Autodesk Inventor part; units mm, degrees
(part 2 of 2)
sketch "スケッチ6" plane through (0, 0, 0) normal (0, 0, 1) x (1, 0, 0)
  arc A0 (-3.1442, 14.278) -> (-3.8445, 14.3466) centre (-3.5856, 13.3807) ccw projected
  arc A1 (-3.8445, 14.3466) -> (-4.7248, 14.0812) centre (0, 0) ccw projected
  arc A2 (-5.6301, 14.2199) -> (-4.7248, 14.0812) centre (-5.0429, 15.0293) ccw projected
  arc A3 (-5.6301, 14.2199) -> (-11.7841, 9.7488) centre (-7.979, 10.9821) ccw projected
  arc A4 (-11.932, 8.8449) -> (-11.7841, 9.7488) centre (-12.7354, 9.4404) ccw projected
  arc A5 (-11.932, 8.8449) -> (-12.4564, 8.0897) centre (0, 0) ccw projected
  arc A6 (-12.4564, 8.0897) -> (-12.6076, 7.4025) centre (-11.6178, 7.545) ccw projected
  arc A7 (-12.6076, 7.4025) -> (-11.6883, 4.5478) centre (-3.7583, 8.6769) ccw projected
  arc A8 (-12.1291, 3.191) -> (-11.6883, 4.5478) centre (-12.5752, 4.0859) ccw projected
  arc A9 (-12.1291, 3.191) -> (-14.5508, 1.4218) centre (-8.1406, -4.8107) ccw projected
  arc A10 (-14.5508, 1.4218) -> (-14.8325, 0.777) centre (-13.8338, 0.7247) ccw projected
  arc A11 (-14.8325, 0.777) -> (-14.8521, -0.1422) centre (0, 0) ccw projected
  arc A12 (-15.2637, -0.9604) -> (-14.8521, -0.1422) centre (-15.8521, -0.1518) ccw projected
  arc A13 (-15.2637, -0.9604) -> (-12.9131, -8.1948) centre (-12.9103, -4.1948) ccw projected
  arc A14 (-12.0992, -8.6148) -> (-12.9131, -8.1948) centre (-12.9138, -9.1948) ccw projected
  arc A15 (-12.0992, -8.6148) -> (-11.543, -9.3469) centre (0, 0) ccw projected
  arc A16 (-11.543, -9.3469) -> (-10.9361, -9.703) centre (-10.7658, -8.7176) ccw projected
  arc A17 (-10.9361, -9.703) -> (-7.9371, -9.7108) centre (-9.4136, -0.893) ccw projected
  arc A18 (-6.7829, -10.5494) -> (-7.9371, -9.7108) centre (-7.7719, -10.6971) ccw projected
  arc A19 (-6.7829, -10.5494) -> (-5.8487, -13.3993) centre (2.0596, -9.2288) ccw projected
  arc A20 (-5.8487, -13.3993) -> (-5.3225, -13.8664) centre (-4.9641, -12.9328) ccw projected
  arc A21 (-5.3225, -13.8664) -> (-4.4543, -14.1692) centre (0, 0) ccw projected
  arc A22 (-3.8033, -14.8134) -> (-4.4543, -14.1692) centre (-4.7542, -15.1231) ccw projected
  arc A23 (-3.8033, -14.8134) -> (3.8033, -14.8134) centre (0, -13.5747) ccw projected
  arc A24 (4.4543, -14.1692) -> (3.8033, -14.8134) centre (4.7542, -15.1231) ccw projected
  arc A25 (4.4543, -14.1692) -> (5.3225, -13.8664) centre (0, 0) ccw projected
  arc A26 (5.3225, -13.8664) -> (5.8487, -13.3993) centre (4.9641, -12.9328) ccw projected
  arc A27 (5.8487, -13.3993) -> (6.7829, -10.5494) centre (-2.0596, -9.2288) ccw projected
  arc A28 (7.9371, -9.7108) -> (6.7829, -10.5494) centre (7.7719, -10.6971) ccw projected
  arc A29 (7.9371, -9.7108) -> (10.9361, -9.703) centre (9.4136, -0.893) ccw projected
  arc A30 (10.9361, -9.703) -> (11.543, -9.3469) centre (10.7658, -8.7176) ccw projected
  arc A31 (11.543, -9.3469) -> (12.0992, -8.6148) centre (0, 0) ccw projected
  arc A32 (12.9131, -8.1948) -> (12.0992, -8.6148) centre (12.9138, -9.1948) ccw projected
  arc A33 (12.9131, -8.1948) -> (15.2637, -0.9604) centre (12.9103, -4.1948) ccw projected
  arc A34 (14.8521, -0.1422) -> (15.2637, -0.9604) centre (15.8521, -0.1518) ccw projected
  arc A35 (14.8521, -0.1422) -> (14.8325, 0.777) centre (0, 0) ccw projected
  arc A36 (14.8325, 0.777) -> (14.5508, 1.4218) centre (13.8338, 0.7247) ccw projected
  arc A37 (14.5508, 1.4218) -> (12.1291, 3.191) centre (8.1406, -4.8107) ccw projected
  arc A38 (11.6883, 4.5478) -> (12.1291, 3.191) centre (12.5752, 4.0859) ccw projected
  arc A39 (11.6883, 4.5478) -> (12.6076, 7.4025) centre (3.7583, 8.6769) ccw projected
  arc A40 (12.6076, 7.4025) -> (12.4564, 8.0897) centre (11.6178, 7.545) ccw projected
  arc A41 (12.4564, 8.0897) -> (11.932, 8.8449) centre (0, 0) ccw projected
  arc A42 (11.7841, 9.7488) -> (11.932, 8.8449) centre (12.7354, 9.4404) ccw projected
  arc A43 (11.7841, 9.7488) -> (5.6301, 14.2199) centre (7.979, 10.9821) ccw projected
  arc A44 (4.7248, 14.0812) -> (5.6301, 14.2199) centre (5.0429, 15.0293) ccw projected
  arc A45 (4.7248, 14.0812) -> (3.8445, 14.3466) centre (0, 0) ccw projected
  arc A46 (3.8445, 14.3466) -> (3.1442, 14.278) centre (3.5856, 13.3807) ccw projected
  arc A47 (3.1442, 14.278) -> (0.7133, 12.5215) centre (7.0908, 6.2556) ccw projected
  arc A48 (-0.7133, 12.5215) -> (0.7133, 12.5215) centre (0, 13.2224) ccw projected
  arc A49 (-0.7133, 12.5215) -> (-3.1442, 14.278) centre (-7.0908, 6.2556) ccw projected
  circle A50 centre (0, 0) radius 3 projected
  circle A51 centre (7.979, 10.9821) radius 1.25 projected
  circle A52 centre (0, -13.5747) radius 1.25 projected
  circle A53 centre (-12.9103, -4.1948) radius 1.25 projected
  circle A54 centre (12.9103, -4.1948) radius 1.25 projected
  circle A55 centre (-7.979, 10.9821) radius 1.25 projected
  arc A56 (-23.736, 0.815) -> (-23.6527, 2.1471) centre (0, 0) ccw
  arc A57 (-28.548, 3.4019) -> (-28.6315, 2.6079) centre (0, 0) ccw projected
  arc A58 (-23.6527, 2.1471) -> (-23.736, 0.815) centre (0, 0) ccw
  line L0 (-13.9599, 19.2142) -> (13.9599, -19.2142) construction
  line L1 (-15.9824, 17.7447) -> (11.9374, -20.6836)
  line L2 (15.9824, -17.7447) -> (-11.9374, 20.6836)
  arc A59 (-11.9374, 20.6836) -> (-15.9824, 17.7447) centre (-13.9599, 19.2142) ccw construction
  arc A60 (11.9374, -20.6836) -> (15.9824, -17.7447) centre (13.9599, -19.2142) ccw construction
  line L3 (-21.815, -9.7168) -> (23.3601, 4.9615)
  line L4 (21.815, 9.7168) -> (-23.3601, -4.9615)
  line L5 (2.5, -23.75) -> (2.5, 23.75)
  line L6 (-2.5, 23.75) -> (-2.5, -23.75)
  line L7 (23.3601, -4.9615) -> (-21.815, 9.7168)
  line L8 (-23.3601, 4.9615) -> (21.815, -9.7168)
  line L9 (11.9374, 20.6836) -> (-15.9824, -17.7447)
  line L10 (-11.9374, -20.6836) -> (15.9824, 17.7447)
  arc A61 (-17.8358, 0.7791) -> (-13.9715, -11.1139) centre (-12.9103, -4.1948) ccw
  arc A62 (-17.8283, 0.934) -> (-17.8358, 0.7791) centre (0, 0) ccw
  arc A63 (-16.7017, 3.5131) -> (-17.8283, 0.934) centre (-13.8338, 0.7247) ccw
  arc A64 (-15.0864, 4.9019) -> (-16.7017, 3.5131) centre (-8.1406, -4.8107) ccw
  arc A65 (-15.5769, 6.9749) -> (-15.0864, 4.9019) centre (-3.7583, 8.6769) ccw
  arc A66 (-14.9724, 9.7236) -> (-15.5769, 6.9749) centre (-11.6178, 7.545) ccw
  arc A67 (-14.8874, 9.8533) -> (-14.9724, 9.7236) centre (0, 0) ccw
  arc A68 (-4.7706, 17.2036) -> (-14.8874, 9.8533) centre (-7.979, 10.9821) ccw
  arc A69 (-4.621, 17.2444) -> (-4.7706, 17.2036) centre (0, 0) ccw
  arc A70 (-1.8199, 16.9699) -> (-4.621, 17.2444) centre (-3.5856, 13.3807) ccw
  arc A71 (0, 15.8628) -> (-1.8199, 16.9699) centre (-7.0908, 6.2556) ccw
  arc A72 (1.8199, 16.9699) -> (0, 15.8628) centre (7.0908, 6.2556) ccw
  arc A73 (4.621, 17.2444) -> (1.8199, 16.9699) centre (3.5856, 13.3807) ccw
  arc A74 (4.7706, 17.2036) -> (4.621, 17.2444) centre (0, 0) ccw
  arc A75 (14.8874, 9.8533) -> (4.7706, 17.2036) centre (7.979, 10.9821) ccw
  arc A76 (14.9724, 9.7236) -> (14.8874, 9.8533) centre (0, 0) ccw
  arc A77 (15.5769, 6.9749) -> (14.9724, 9.7236) centre (11.6178, 7.545) ccw
  arc A78 (15.0864, 4.9019) -> (15.5769, 6.9749) centre (3.7583, 8.6769) ccw
  arc A79 (16.7017, 3.5131) -> (15.0864, 4.9019) centre (8.1406, -4.8107) ccw
  arc A80 (17.8283, 0.934) -> (16.7017, 3.5131) centre (13.8338, 0.7247) ccw
  arc A81 (17.8358, 0.7791) -> (17.8283, 0.934) centre (0, 0) ccw
  arc A82 (13.9715, -11.1139) -> (17.8358, 0.7791) centre (12.9103, -4.1948) ccw
  arc A83 (13.8745, -11.2348) -> (13.9715, -11.1139) centre (0, 0) ccw
  arc A84 (11.447, -12.6592) -> (13.8745, -11.2348) centre (10.7658, -8.7176) ccw
  arc A85 (9.3239, -12.8333) -> (11.447, -12.6592) centre (9.4136, -0.893) ccw
  arc A86 (8.5023, -14.7987) -> (9.3239, -12.8333) centre (-2.0596, -9.2288) ccw
  arc A87 (6.3975, -16.6672) -> (8.5023, -14.7987) centre (4.9641, -12.9328) ccw
  arc A88 (6.2525, -16.7221) -> (6.3975, -16.6672) centre (0, 0) ccw
  arc A89 (-6.2525, -16.7221) -> (6.2525, -16.7221) centre (0, -13.5747) ccw
  arc A90 (-6.3975, -16.6672) -> (-6.2525, -16.7221) centre (0, 0) ccw
  arc A91 (-8.5023, -14.7987) -> (-6.3975, -16.6672) centre (-4.9641, -12.9328) ccw
  arc A92 (-9.3239, -12.8333) -> (-8.5023, -14.7987) centre (2.0596, -9.2288) ccw
  arc A93 (-11.447, -12.6592) -> (-9.3239, -12.8333) centre (-9.4136, -0.893) ccw
  arc A94 (-13.8745, -11.2348) -> (-11.447, -12.6592) centre (-10.7658, -8.7176) ccw
  arc A95 (-13.9715, -11.1139) -> (-13.8745, -11.2348) centre (0, 0) ccw
  point P0 (-2.5, 13.9276)
  point P1 (-2.5, 23.6181)
  point P2 (-11.8598, 20.5769)
  point P3 (-7.7918, 14.9777)
  point P4 (7.7918, 14.9777)
  point P5 (11.8598, 20.5769)
  point P6 (2.5, 23.6181)
  point P7 (2.5, 13.9276)
  point P8 (-11.8369, 12.0388)
  point P9 (-15.9049, 17.6379)
  point P10 (-21.6896, 9.676)
  point P11 (-12.4733, 6.6815)
  point P12 (-14.0184, 1.9262)
  point P13 (-23.2346, 4.9207)
  point P14 (-23.2346, -4.9207)
  point P15 (-16.6525, -2.7821)
  point P16 (-15.1074, -7.5373)
  point P17 (-21.6896, -9.676)
  point P18 (-15.9049, -17.6379)
  point P19 (-10.209, -9.7982)
  point P20 (-6.1639, -12.7371)
  point P21 (-11.8598, -20.5769)
  point P22 (-2.5, -23.6181)
  point P23 (-2.5, -16.6972)
  point P24 (2.5, -16.6972)
  point P25 (2.5, -23.6181)
  point P26 (11.8598, -20.5769)
  point P27 (6.1639, -12.7371)
  point P28 (10.209, -9.7982)
  point P29 (15.9049, -17.6379)
  point P30 (21.6896, -9.676)
  point P31 (15.1074, -7.5373)
  point P32 (16.6525, -2.7821)
  point P33 (23.2346, -4.9207)
  point P34 (23.2346, 4.9207)
  point P35 (14.0184, 1.9262)
  point P36 (12.4733, 6.6815)
  point P37 (21.6896, 9.676)
  point P38 (15.9049, 17.6379)
  point P39 (11.8369, 12.0388)
  point P40 (15.6147, 7.7022)
  point P41 (13.8447, 14.8023)
  point P42 (19.9012, -3.8376)
  point P43 (17.1598, 2.9469)
  point P44 (12.1504, -12.4703)
  point P45 (18.3561, -8.5929)
  point P46 (2.5, -20.113)
  point P47 (8.1053, -15.4093)
  point P48 (-8.1053, -15.4093)
  point P49 (-2.5, -20.113)
  point P50 (-18.3561, -8.5929)
  point P51 (-12.1504, -12.4703)
  point P52 (-19.9012, -3.8376)
  point P53 (-17.1598, 2.9469)
  point P54 (-13.8447, 14.8023)
  point P55 (-15.6147, 7.7022)
  point P56 (9.7996, 17.7412)
  point P57 (2.5, 17.2306)
  point P58 (-2.5, 17.2306)
  point P59 (-9.7996, 17.7412)
  dimension "d16" = 5
  dimension "d17" = 5
  dimension "d20" = 360
  dimension "d24" = 3
  constraints: 79 point on circle, 39 centre point, 24 end point, 4 tangent, 2 concentric, 1 coincident, 1 midpoint, 1 parallel, 1 point on line, 65 other
  measures "d16" radial gap between concentric circles of A56 A57
  measures "d17" diameter of A60
  measures "d24" radial gap between concentric circles of A13 A61
extrude "押し出し4" cut sketch "スケッチ6" against normal through all contours A70 A69 A68 L2 A56 L6 | A56 L9 A75 A74 A73 L5 | L1 A68 A67 A66 L7 A56 | L2 L7 L4 A50 | A50 L7 L2 | L4 L7 A50 | L7 L4 L9 A50 | L9 L4 A50 | L4 L9 L6 A50 | L6 L9 A50 | A56 L4 A77 A76 A75 L10 | A50 L5 L2 L7 | L2 L5 L10 L3 L8 L1 L6 L9 L4 L7 | L9 L6 L1 A50 | L8 A63 A62 A61 L4 A56 A58 | A50 L2 L5 | L2 A50 L10 L5 | L1 L6 A50 | L1 L8 A50 L6 | A56 L7 A82 A81 A80 L3 | L10 A50 L5 | L5 A50 L3 L10 | L8 L3 A50 L1 | L1 A50 L8 | L10 A50 L8 L3 | L3 A50 L10 | A61 A95 A94 L9 A56 L3 | L8 A50 L3 | A56 L2 A84 A83 A82 L8 | A56 L5 A89 A88 A87 L1 | L6 A56 L10 A91 A90 A89 | A51 | A52 | A53 | A54 | A55
fillet "フィレット3" radius 1 50 edges at (-12.1504, -12.4703, -2.5) (-13.9715, -11.1139, -2.5) (-18.3561, -8.5929, -2.5) (-15.9049, -17.6379, -2.5) (-21.6896, -9.676, -2.5) (-8.1053, -15.4093, -2.5) (-6.2525, -16.7221, -2.5) (-2.5, -20.113, -2.5) (-2.5, -23.6181, -2.5) (11.8598, -20.5769, -2.5) (-11.8598, -20.5769, -2.5) (2.5, -20.113, -2.5) (6.2525, -16.7221, -2.5) (8.1053, -15.4093, -2.5) (18.3561, -8.5929, -2.5) (13.9715, -11.1139, -2.5) (2.5, -23.6181, -2.5) (19.9012, -3.8376, -2.5) (17.8358, 0.7791, -2.5) (14.8874, 9.8533, -2.5) (15.6147, 7.7022, -2.5) (-23.2346, -4.9207, -2.5) (-21.6896, 9.676, -2.5) (-9.7996, 17.7412, -2.5) (-4.7706, 17.2036, -2.5) (2.5, 17.2306, -2.5) (4.7706, 17.2036, -2.5) (13.8447, 14.8023, -2.5) (15.9049, -17.6379, -2.5) (23.2346, -4.9207, -2.5) (-2.5, 17.2306, -2.5) (9.7996, 17.7412, -2.5) (-15.6147, 7.7022, -2.5) (-19.9012, -3.8376, -2.5) (-17.8358, 0.7791, -2.5) (-14.8874, 9.8533, -2.5) (-2.5, 23.6181, -2.5) (11.8598, 20.5769, -2.5) (21.6896, -9.676, -2.5) (23.2346, 4.9207, -2.5) (12.1504, -12.4703, -2.5) (17.1598, 2.9469, -2.5) (2.5, 23.6181, -2.5) (-11.8598, 20.5769, -2.5) (-23.2346, 4.9207, -2.5) (-15.9049, 17.6379, -2.5) (15.9049, 17.6379, -2.5) (21.6896, 9.676, -2.5) (-13.8447, 14.8023, -2.5) (-17.1598, 2.9469, -2.5)
chamfer "面取り1" distance 1.75 angle 45 5 edges at (-9.229, 10.9821, -5) (6.729, 10.9821, -5) (11.6603, -4.1948, -5) (-1.25, -13.5747, -5) (-14.1603, -4.1948, -5)
body "Solid1"
